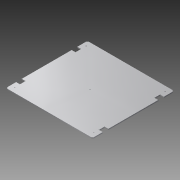
# Autodesk Inventor part: stolik
Saved by Autodesk Inventor 2013 (Build 170138000, 138)
## iProperties
Created: 2013-11-19
Part Number: stolik
Material: Generic
Document SubType Name: Modeling
Designer: Masta
Density: 1 g/cm^3
Author: Masta
Autodesk Inventor part; units mm, degrees
ref_plane "YZ Plane" through (0, 0, 0) normal (1, 0, 0) x (0, 1, 0)
ref_plane "XZ Plane" through (0, 0, 0) normal (0, 1, 0) x (-1, 0, 0)
ref_plane "XY Plane" through (0, 0, 0) normal (0, 0, 1) x (1, 0, 0)
sketch "Sketch1" plane through (0, 0, 0) normal (0, 0, 1) x (1, 0, 0)
  line L0 (-170, -160) -> (170, -160)
  line L1 (170, -160) -> (170, -120)
  line L2 (170, 160) -> (-170, 160)
  line L3 (-170, 160) -> (-170, 120)
  line L4 (-170, -160) -> (170, 160) construction
  line L5 (170, -160) -> (-170, 160) construction
  line L6 (-155, -140) -> (155, -140) construction
  line L7 (155, -140) -> (155, 140) construction
  line L8 (155, 140) -> (-155, 140) construction
  line L9 (-155, 140) -> (-155, -140) construction
  line L10 (-155, -140) -> (155, 140) construction
  line L11 (155, -140) -> (-155, 140) construction
  line L12 (-150, -150) -> (150, -150) construction
  line L13 (150, -150) -> (150, 150) construction
  line L14 (150, 150) -> (-150, 150) construction
  line L15 (-150, 150) -> (-150, -150) construction
  line L16 (-150, -150) -> (150, 150) construction
  line L17 (150, -150) -> (-150, 150) construction
  line L18 (170, 120) -> (155, 120)
  line L19 (155, 120) -> (155, 98)
  line L20 (155, 98) -> (170, 98)
  line L21 (170, 98) -> (170, 120) construction
  line L22 (0, -160) -> (0, 160) construction
  line L23 (-170, 0) -> (170, 0) construction
  line L24 (-170, 120) -> (-155, 120)
  line L25 (-155, 120) -> (-155, 98)
  line L26 (-155, 98) -> (-170, 98)
  line L27 (-170, 98) -> (-170, 120) construction
  line L28 (170, -120) -> (155, -120)
  line L29 (155, -120) -> (155, -98)
  line L30 (155, -98) -> (170, -98)
  line L31 (170, -98) -> (170, -120) construction
  line L32 (-170, -120) -> (-155, -120)
  line L33 (-155, -98) -> (-170, -98)
  line L34 (-170, -98) -> (-170, -120) construction
  line L35 (-155, -120) -> (-155, -98)
  line L36 (-170, 98) -> (-170, -98)
  line L37 (-170, -120) -> (-170, -160)
  line L38 (-170, -98) -> (-170, -120)
  line L39 (170, -120) -> (170, -98)
  line L40 (170, -98) -> (170, 98)
  line L41 (170, 98) -> (170, 120)
  line L42 (170, 120) -> (170, 160)
  line L43 (-170, 120) -> (-170, 98) construction
  point P0 (0, 0)
  point P1 (0, 0)
  dimension "d0" = 340
  dimension "d1" = 320
  dimension "d4" = 310
  dimension "d5" = 280
  dimension "d13" = 300
  dimension "d14" = 300
  dimension "d15" = 22
  dimension "d16" = 30
  constraints: 88 end point, 32 parallel, 12 symmetric about line, 9 midpoint, 8 perpendicular, 5 coincident, 4 horizontal, 4 point on line
  measures "d0" distance of L2.end L2.start
  measures "d1" distance of L2.start L0.end
  measures "d4" distance of L8.end L7.end
  measures "d5" distance of L7.end L6.end
  measures "d13" distance of L14.end L13.end
  measures "d14" distance of L13.end L12.end
  measures "d15" distance of L20.end L18.start
  measures "d16" distance between parallel lines of L14 L18
extrude "Extrusion1" add sketch "Sketch1" along normal blind 4 contours L37 L32 L35 L33 L36 L26 L25 L24 L3 L2 L42 L18 L19 L20 L40 L30 L29 L28 L1 L0
hole "Hole1" at (-155, 140, 0) at (-155, -140, 0) at (155, -140, 0) at (155, 140, 0) at (0, 0, 0) direction (0, 0, 1) diameter 3.2 end through all
sketch "Szkic2" plane through (0, 0, 4) normal (0, 0, 1) x (1, 0, 0)
  point P0 (-155, 98)
  point P1 (-155, 120)
  point P2 (-155, -120)
  point P3 (-155, -98)
  point P4 (155, -120)
  point P5 (155, -98)
  point P6 (155, 98)
  point P7 (155, 120)
hole "Otwór2" at (-155, 98, 4) at (-155, 120, 4) at (-155, -120, 4) at (-155, -98, 4) at (155, -120, 4) at (155, -98, 4) at (155, 98, 4) at (155, 120, 4) direction (0, 0, -1) diameter 1 end through all
chamfer "Faza1" distance 5 angle 45 4 edges at (-170, -160, 2) (170, -160, 2) (170, 160, 2) (-170, 160, 2)
body "Solid1"
